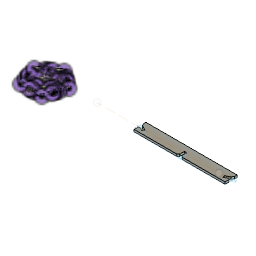
ico-kit (Autodesk Fusion 360 design; units mm, degrees)
part number: 2025-09-22-00-08-37-504
part number: 2025-09-22-13-11-55-627
part number: 2025-09-22-16-05-58-126
Autodesk Fusion 360 part; units mm, degrees
sketch "Sketch1" plane through (0, 0, 0) normal (0, 0, 1) x (1, 0, 0) in component "ico_joint"
  line L0 (0, 12) -> (-11.4127, 3.7082)
  line L1 (-11.4127, 3.7082) -> (-7.0534, -9.7082)
  line L2 (-7.0534, -9.7082) -> (7.0534, -9.7082)
  line L3 (7.0534, -9.7082) -> (11.4127, 3.7082)
  line L4 (11.4127, 3.7082) -> (0, 12)
  line L5 (0, 0) -> (5.7063, 7.8541) construction
  line L6 (0, 0) -> (-5.7063, 7.8541) construction
  line L7 (0, 0) -> (-9.2331, -3) construction
  line L8 (0, 0) -> (0, -9.7082) construction
  line L9 (0, 0) -> (9.2331, -3) construction
  line L10 (3.9215, 4.2066) -> (6.2727, 7.4427)
  line L11 (6.2727, 7.4427) -> (5.14, 8.2656)
  line L12 (5.14, 8.2656) -> (2.7889, 5.0295)
  line L13 (2.7889, 5.0295) -> (3.9215, 4.2066)
  line L14 (9.4494, -2.3343) -> (9.0167, -3.6657)
  line L15 (9.0167, -3.6657) -> (5.2125, -2.4297)
  line L16 (5.2125, -2.4297) -> (5.6451, -1.0982)
  line L17 (5.6451, -1.0982) -> (9.4494, -2.3343)
  line L18 (-6.2727, 7.4427) -> (-3.9215, 4.2066)
  line L19 (-3.9215, 4.2066) -> (-2.7889, 5.0295)
  line L20 (-2.7889, 5.0295) -> (-5.14, 8.2656)
  line L21 (-5.14, 8.2656) -> (-6.2727, 7.4427)
  line L22 (-9.0056, -3.7) -> (-5.2014, -2.4639)
  line L23 (-5.2014, -2.4639) -> (-5.6563, -1.0639)
  line L24 (-5.6563, -1.0639) -> (-9.4605, -2.3)
  line L25 (-9.4605, -2.3) -> (-9.0056, -3.7)
  line L26 (0.7, -5.7082) -> (0.7, -9.7082)
  line L27 (0.7, -9.7082) -> (-0.7, -9.7082)
  line L28 (-0.7, -9.7082) -> (-0.7, -5.7082)
  line L29 (-0.7, -5.7082) -> (0.7, -5.7082)
  line L30 (0.7, -9.7082) -> (0.8, -9.7082)
  line L31 (0.8, -9.7082) -> (0.8, -9.6082) construction
  line L32 (0.8, -9.6082) -> (0.7, -9.6082) construction
  line L33 (0.7, -9.6082) -> (0.7, -9.7082)
  line L34 (-0.7, -9.7082) -> (-0.8, -9.7082)
  line L35 (-0.8, -9.7082) -> (-0.8, -9.6082) construction
  line L36 (-0.8, -9.6082) -> (-0.7, -9.6082) construction
  line L37 (-0.7, -9.6082) -> (-0.7, -9.7082)
  arc A0 (-0.8, -9.7082) -> (-0.7, -9.6082) centre (-0.8, -9.6082) ccw
  line L38 (-9.4605, -2.3) -> (-9.4914, -2.2049)
  line L39 (-9.4914, -2.2049) -> (-9.3963, -2.174) construction
  line L40 (-9.3963, -2.174) -> (-9.3654, -2.2691) construction
  line L41 (-9.3654, -2.2691) -> (-9.4605, -2.3)
  line L42 (-9.0056, -3.7) -> (-8.9747, -3.7951)
  line L43 (-8.9747, -3.7951) -> (-8.8796, -3.7642) construction
  line L44 (-8.8796, -3.7642) -> (-8.9105, -3.6691) construction
  line L45 (-8.9105, -3.6691) -> (-9.0056, -3.7)
  line L46 (-6.2727, 7.4427) -> (-6.3536, 7.3839)
  line L47 (-6.3536, 7.3839) -> (-6.2948, 7.303) construction
  line L48 (-6.2948, 7.303) -> (-6.2139, 7.3618) construction
  line L49 (-6.2139, 7.3618) -> (-6.2727, 7.4427)
  line L50 (-5.14, 8.2656) -> (-5.0591, 8.3243)
  line L51 (-5.0591, 8.3243) -> (-5.0003, 8.2434) construction
  line L52 (-5.0003, 8.2434) -> (-5.0812, 8.1846) construction
  line L53 (-5.0812, 8.1846) -> (-5.14, 8.2656)
  line L54 (9.0167, -3.6657) -> (8.9858, -3.7608)
  line L55 (8.9858, -3.7608) -> (8.8907, -3.7299) construction
  line L56 (8.8907, -3.7299) -> (8.9216, -3.6348) construction
  line L57 (8.9216, -3.6348) -> (9.0167, -3.6657)
  line L58 (9.4494, -2.3343) -> (9.4803, -2.2392)
  line L59 (9.4803, -2.2392) -> (9.3852, -2.2083) construction
  line L60 (9.3852, -2.2083) -> (9.3543, -2.3034) construction
  line L61 (9.3543, -2.3034) -> (9.4494, -2.3343)
  line L62 (6.2727, 7.4427) -> (6.3536, 7.3839)
  line L63 (6.3536, 7.3839) -> (6.2948, 7.303) construction
  line L64 (6.2948, 7.303) -> (6.2139, 7.3618) construction
  line L65 (6.2139, 7.3618) -> (6.2727, 7.4427)
  line L66 (5.14, 8.2656) -> (5.0591, 8.3243)
  line L67 (5.0591, 8.3243) -> (5.0003, 8.2434) construction
  line L68 (5.0003, 8.2434) -> (5.0812, 8.1846) construction
  line L69 (5.0812, 8.1846) -> (5.14, 8.2656)
  arc A1 (-8.9105, -3.6691) -> (-8.9747, -3.7951) centre (-8.8796, -3.7642) ccw
  arc A2 (-9.4914, -2.2049) -> (-9.3654, -2.2691) centre (-9.3963, -2.174) ccw
  arc A3 (-6.2139, 7.3618) -> (-6.3536, 7.3839) centre (-6.2948, 7.303) ccw
  arc A4 (-5.0591, 8.3243) -> (-5.0812, 8.1846) centre (-5.0003, 8.2434) ccw
  arc A5 (5.0812, 8.1846) -> (5.0591, 8.3243) centre (5.0003, 8.2434) ccw
  arc A6 (9.3543, -2.3034) -> (9.4803, -2.2392) centre (9.3852, -2.2083) ccw
  arc A7 (8.9858, -3.7608) -> (8.9216, -3.6348) centre (8.8907, -3.7299) ccw
  line L70 (-2.7889, 5.0295) -> (-3.9215, 4.2066)
  line L71 (-3.9215, 4.2066) -> (-1.5704, 0.9705) construction
  line L72 (-1.5704, 0.9705) -> (-0.4377, 1.7934) construction
  line L73 (-0.4377, 1.7934) -> (-2.7889, 5.0295) construction
  line L74 (3.9215, 4.2066) -> (2.7889, 5.0295)
  line L75 (2.7889, 5.0295) -> (0.4377, 1.7934) construction
  line L76 (0.4377, 1.7934) -> (1.5704, 0.9705) construction
  line L77 (1.5704, 0.9705) -> (3.9215, 4.2066) construction
  arc A8 (6.3536, 7.3839) -> (6.2139, 7.3618) centre (6.2948, 7.303) ccw
  arc A9 (0.7, -9.6082) -> (0.8, -9.7082) centre (-0.2726, -10.6808) ccw construction
  dimension "d6" = 12
  dimension "d14" = 4
  dimension "d15" = 1.4
  dimension "d16" = 1.4
  dimension "d17" = 4
  dimension "d18" = 4
  dimension "d19" = 1.4
  dimension "d20" = 4
  dimension "d21" = 1.4
  dimension "d22" = 4
  dimension "d23" = 1.4
  dimension "d27" = 0.1
  dimension "d28" = 0.1
  dimension "d29" = 0.1
  dimension "d30" = 0.1
  dimension "d31" = 0.1
  dimension "d32" = 0.1
  dimension "d33" = 0.1
  dimension "d34" = 0.1
  dimension "d35" = 0.1
  dimension "d36" = 0.1
  dimension "d37" = 0.1
  dimension "d38" = 4
  dimension "d39" = 4
  constraint coincident L5.start L6.start
  constraint midpoint L4 L5.end
  constraint midpoint L0 L6.end
  constraint midpoint L1 L7.end
  constraint midpoint L2 L8.end
  constraint midpoint L3 L9.end
  constraint perpendicular L10 L11
  constraint parallel L10 L12
  constraint parallel L11 L13
  constraint perpendicular L4 L12
  constraint midpoint L4 L11
  constraint perpendicular L14 L15
  constraint parallel L14 L16
  constraint parallel L15 L17
  constraint perpendicular L3 L17
  constraint midpoint L3 L14
  constraint perpendicular L18 L19
  constraint parallel L18 L20
  constraint parallel L19 L21
  constraint perpendicular L0 L20
  constraint midpoint L0 L21
  constraint perpendicular L22 L23
  constraint parallel L22 L24
  constraint parallel L23 L25
  constraint midpoint L1 L25
  constraint perpendicular L1 L24
  constraint perpendicular L26 L27
  constraint parallel L26 L28
  constraint parallel L27 L29
  constraint vertical L26
  constraint perpendicular L2 L28
  constraint midpoint L2 L27
  constraint perpendicular L30 L31
  constraint parallel L30 L32
  constraint parallel L31 L33
  constraint perpendicular L26 L30
  constraint perpendicular L34 L35
  constraint parallel L34 L36
  constraint parallel L35 L37
  constraint perpendicular L28 L34
  constraint coincident L35.end L36.start
  constraint perpendicular L38 L39
  constraint parallel L38 L40
  constraint parallel L39 L41
  constraint perpendicular L24 L38
  constraint perpendicular L42 L43
  constraint parallel L42 L44
  constraint parallel L43 L45
  constraint perpendicular L22 L42
  constraint perpendicular L46 L47
  constraint parallel L46 L48
  constraint parallel L47 L49
  constraint perpendicular L18 L46
  constraint perpendicular L50 L51
  constraint parallel L50 L52
  constraint parallel L51 L53
  constraint perpendicular L20 L50
  constraint perpendicular L54 L55
  constraint parallel L54 L56
  constraint parallel L55 L57
  constraint perpendicular L15 L54
  constraint perpendicular L58 L59
  constraint parallel L58 L60
  constraint parallel L59 L61
  constraint perpendicular L17 L58
  constraint perpendicular L62 L63
  constraint parallel L62 L64
  constraint parallel L63 L65
  constraint perpendicular L10 L62
  constraint perpendicular L66 L67
  constraint parallel L66 L68
  constraint parallel L67 L69
  constraint perpendicular L12 L66
  constraint coincident L43.end L44.start
  constraint coincident L39.end L40.start
  constraint coincident L47.end L48.start
  constraint coincident L51.end L52.start
  constraint coincident L67.end L68.start
  constraint coincident L59.end L60.start
  constraint coincident L55.end L56.start
  constraint perpendicular L70 L71
  constraint parallel L70 L72
  constraint parallel L71 L73
  constraint perpendicular L74 L75
  constraint parallel L74 L76
  constraint parallel L75 L77
  constraint coincident L63.end L64.start
  measures "d6" distance of L0.start L5.start
  measures "d14" distance of L10.start L10.end
  measures "d15" distance of L10.start L12.end
  measures "d16" distance of L14.start L14.end
  measures "d17" distance of L14.start L16.end
  measures "d18" distance of L18.start L18.end
  measures "d19" distance of L18.start L20.end
  measures "d20" distance of L22.start L22.end
  measures "d21" vertical distance of L22.end L23.end
  measures "d22" distance of L27.end L28.end
  measures "d23" distance of L26.start L28.end
  measures "d27" distance of L26.end L30.end
  measures "d28" distance of L26.end L32.end
  measures "d29" distance of L27.end L36.end
  measures "d30" distance of L24.end L40.end
  measures "d31" distance of L22.start L44.end
  measures "d32" distance of L18.start L48.end
  measures "d33" distance of L20.end L52.end
  measures "d34" distance of L14.end L56.end
  measures "d35" distance of L14.start L60.end
  measures "d36" distance of L10.end L64.end
  measures "d37" distance of L11.end L68.end
  measures "d38" distance of L19.end L72.end
  measures "d39" distance of L10.start L76.end
sketch "Sketch1 (2)" plane through (0, 0, 0) normal (0, 0, 1) x (1, 0, 0) in component "ico_beam"
  line L0 (57.3604, 0.4256) -> (117.3604, 0.4256)
  line L1 (117.3604, 0.4256) -> (117.3604, 8.4256)
  line L2 (117.3604, 8.4256) -> (57.3604, 8.4256)
  line L3 (57.3604, 8.4256) -> (57.3604, 0.4256)
  line L4 (57.3604, 4.8668) -> (60.9307, 3.0633) construction
  line L5 (57.3604, 4.8668) -> (28.6971, 4.8668) construction
  line L6 (57.3604, 4.8668) -> (117.3604, 4.8668) construction
  line L7 (117.3604, 4.8668) -> (113.79, 3.0633) construction
  line L8 (117.3604, 4.8668) -> (109, 4.8668) construction
  line L9 (55.8908, 6.3934) -> (61.2463, 3.6881)
  line L10 (61.2463, 3.6881) -> (60.6151, 2.4385)
  line L11 (60.6151, 2.4385) -> (55.2596, 5.1438)
  line L12 (55.2596, 5.1438) -> (55.8908, 6.3934)
  line L13 (114.1056, 2.4385) -> (119.4611, 5.1438)
  line L14 (119.4611, 5.1438) -> (118.8299, 6.3934)
  line L15 (118.8299, 6.3934) -> (113.4744, 3.6881)
  line L16 (113.4744, 3.6881) -> (114.1056, 2.4385)
  line L17 (86.6604, 4.4256) -> (86.6604, 0.4256)
  line L18 (86.6604, 0.4256) -> (88.0604, 0.4256)
  line L19 (88.0604, 0.4256) -> (88.0604, 4.4256)
  line L20 (88.0604, 4.4256) -> (86.6604, 4.4256)
  dimension "d49" = 60
  dimension "d50" = 8
  dimension "d51" = 26.8
  dimension "d52" = 4
  dimension "d53" = 153.2
  dimension "d54" = 4
  dimension "d55" = 6
  dimension "d56" = 1.4
  dimension "d57" = 6
  dimension "d58" = 1.4
  dimension "d63" = 4
  dimension "d64" = 1.4
  constraint horizontal L0
  constraint vertical L1
  constraint horizontal L2
  constraint vertical L3
  constraint horizontal L5
  constraint perpendicular L1 L6
  constraint horizontal L8
  constraint perpendicular L9 L10
  constraint parallel L9 L11
  constraint parallel L10 L12
  constraint parallel L4 L9
  constraint midpoint L4.end L10
  constraint coincident L3 L4.start
  constraint perpendicular L13 L14
  constraint parallel L13 L15
  constraint parallel L14 L16
  constraint parallel L7 L15
  constraint midpoint L7.end L16
  constraint coincident L1 L6.end
  constraint perpendicular L17 L18
  constraint parallel L17 L19
  constraint parallel L18 L20
  constraint perpendicular L2 L17
  constraint midpoint L0 L18
  measures "d49" distance of L0.start L0.end
  measures "d50" distance of L0.start L2.end
  measures "d51" angle of L4 L5
  measures "d52" distance of L4.start L4.end
  measures "d53" angle of L7 L8
  measures "d54" distance of L6.end L7.end
  measures "d55" distance of L9.start L9.end
  measures "d56" distance of L9.start L11.end
  measures "d57" distance of L13.start L13.end
  measures "d58" distance of L13.start L15.end
  measures "d63" distance of L17.start L17.end
  measures "d64" distance of L17.start L19.end
extrude "Extrude3" add sketch "Sketch1 (2)" along normal blind 1.4 contours L0 L1 L2 L3 L9 L10 L11 L13 L15 L16 L17 L19 L20 makes body 1 in component "ico_beam"
extrude "Extrude4" add sketch "Sketch1" along normal blind 1.4 separate body contours L0 L1 L2 L3 L4 L10 L12 L13 L15 L16 L17 L18 L19 L20 L22 L23 L24 L26 L28 L29 L30 L33 A0 A1 A2 A3 A4 A5 A6 A7 L70 L74 A8 | L0 L20 L50 L53 A4 | L4 L12 L66 L69 A5 | L0 L18 L46 L49 A3 | L4 L10 L62 L65 A8 | L1 L24 L38 L41 A2 | L3 L17 L58 L61 A6 | L1 L22 L42 L45 A1 | L3 L15 L54 L57 A7 | L2 L28 L34 L37 A0 makes body 2 in component "ico_joint"
chamfer "Chamfer1" distance 1 angle 45 4 edges at (9.0167, -3.6657, 0.7) (9.4494, -2.3343, 0.7) (5.14, 8.2656, 0.7) (6.2727, 7.4427, 0.7) on bodies 2 in component "ico_joint"
chamfer "Chamfer2" distance 1 angle 45 4 edges at (-5.14, 8.2656, 0.7) (-6.2727, 7.4427, 0.7) (-9.0056, -3.7, 0.7) (-0.7, -9.7082, 0.7) on bodies 2 in component "ico_joint"
chamfer "Chamfer3" distance 1 angle 45 2 edges at (-9.4605, -2.3, 0.7) (0.7, -9.7082, 0.7) on bodies 2 in component "ico_joint"
chamfer "Chamfer1'" distance 1 angle 45 5 edges at (57.3604, 5.6511, 0.7) (57.3604, 4.0826, 0.7) (88.0604, 0.4256, 0.7) (86.6604, 0.4256, 0.7) (117.3604, 5.6511, 0.7) on bodies 1 in component "ico_beam"
chamfer "Chamfer2'" distance 1 angle 45 1 edges at (117.3604, 4.0826, 0.7) on bodies 1 in component "ico_beam"
sketch "Sketch7" plane through (0, 0, 0) normal (0, 0, 1) x (1, 0, 0)
  line L0 (0.7, -8.7082) -> (1.7, -9.7082)
  line L1 (1.7, -9.7082) -> (7.0534, -9.7082)
  line L2 (0.7, -5.7082) -> (0.7, -8.7082)
  line L3 (-0.7, -5.7082) -> (0.7, -5.7082)
  line L4 (-0.7, -8.7082) -> (-0.7, -5.7082)
  line L5 (-1.7, -9.7082) -> (-0.7, -8.7082)
  line L6 (-7.0534, -9.7082) -> (-1.7, -9.7082)
  line L7 (-8.6966, -4.6511) -> (-7.0534, -9.7082)
  line L8 (-8.0546, -3.391) -> (-8.6966, -4.6511)
  line L9 (-8.0546, -3.391) -> (-5.2014, -2.4639)
  line L10 (-5.2014, -2.4639) -> (-5.6563, -1.0639)
  line L11 (-5.6563, -1.0639) -> (-8.5094, -1.991)
  line L12 (-9.7695, -1.3489) -> (-8.5094, -1.991)
  line L13 (-11.4127, 3.7082) -> (-9.7695, -1.3489)
  line L14 (-7.0817, 6.8549) -> (-11.4127, 3.7082)
  line L15 (-5.6849, 6.6336) -> (-7.0817, 6.8549)
  line L16 (-5.6849, 6.6336) -> (-3.9215, 4.2066)
  line L17 (-2.7889, 5.0295) -> (-3.9215, 4.2066)
  line L18 (-2.7889, 5.0295) -> (-4.5522, 7.4565)
  line L19 (-4.331, 8.8533) -> (-4.5522, 7.4565)
  line L20 (0, 12) -> (-4.331, 8.8533)
  line L21 (4.331, 8.8533) -> (0, 12)
  line L22 (4.5522, 7.4565) -> (4.331, 8.8533)
  line L23 (4.5522, 7.4565) -> (2.7889, 5.0295)
  line L24 (3.9215, 4.2066) -> (2.7889, 5.0295)
  line L25 (3.9215, 4.2066) -> (5.6849, 6.6336)
  line L26 (7.0817, 6.8549) -> (5.6849, 6.6336)
  line L27 (11.4127, 3.7082) -> (7.0817, 6.8549)
  line L28 (9.7584, -1.3832) -> (11.4127, 3.7082)
  line L29 (8.4983, -2.0252) -> (9.7584, -1.3832)
  line L30 (5.6451, -1.0982) -> (8.4983, -2.0252)
  line L31 (5.2125, -2.4297) -> (5.6451, -1.0982)
  line L32 (8.0657, -3.3567) -> (5.2125, -2.4297)
  line L33 (8.7077, -4.6168) -> (8.0657, -3.3567)
  line L34 (7.0534, -9.7082) -> (8.7077, -4.6168)
component "ico_joint" placed x (1, 0, 0) y (0, 1, 0) z (0, 0, 1) at (0, 0, 0)
component "ico_beam" placed x (1, 0, 0) y (0, 1, 0) z (0, 0, 1) at (0, 0, 0)
equation "cardboard_joint_width = 1.4 mm"
equation "ico_joint_adius = 12 mm"
equation "d6 = ico_joint_adius"
equation "cardboard_joint_length = 4 mm"
equation "d14 = cardboard_joint_length"
equation "d15 = cardboard_joint_width"
equation "d16 = cardboard_joint_width"
equation "d17 = cardboard_joint_length"
equation "d18 = cardboard_joint_length"
equation "d19 = cardboard_joint_width"
equation "d20 = cardboard_joint_length"
equation "d21 = cardboard_joint_width"
equation "d22 = cardboard_joint_length"
equation "d23 = cardboard_joint_width"
equation "cardboard_joint_miter_radius = 0.1 mm"
equation "d27 = cardboard_joint_miter_radius"
equation "d28 = cardboard_joint_miter_radius"
equation "d29 = cardboard_joint_miter_radius"
equation "d30 = cardboard_joint_miter_radius"
equation "d31 = cardboard_joint_miter_radius"
equation "d32 = cardboard_joint_miter_radius"
equation "d33 = cardboard_joint_miter_radius"
equation "d34 = cardboard_joint_miter_radius"
equation "d35 = cardboard_joint_miter_radius"
equation "d36 = cardboard_joint_miter_radius"
equation "d37 = cardboard_joint_miter_radius"
equation "d38 = cardboard_joint_length"
equation "d39 = cardboard_joint_length"
equation "cardboard_thickness = 1.4 mm"
equation "ico_dihedral_angle = 138.190 deg"
equation "ico_beam_joint_angle = 26.8 deg"
equation "ico_beam_width = 8 mm"
equation "ico_beam_length = 60 mm"
equation "d49 = ico_beam_length"
equation "d50 = ico_beam_width"
equation "d51 = ico_beam_joint_angle"
equation "d52 = cardboard_joint_length"
equation "d53 = 180 deg - ico_beam_joint_angle"
equation "d54 = cardboard_joint_length"
equation "d55 = cardboard_joint_length * 1.5"
equation "d56 = cardboard_joint_width"
equation "d57 = cardboard_joint_length * 1.5"
equation "d58 = cardboard_joint_width"
equation "d63 = cardboard_joint_length"
equation "d64 = cardboard_joint_width"
equation "d65 = cardboard_thickness"
equation "d67 = cardboard_thickness"
equation "chamfer = 1 mm"
equation "d70 = chamfer"
equation "d71 = chamfer"
equation "d72 = chamfer"
equation "d73 = chamfer"
equation "d74 = chamfer"
